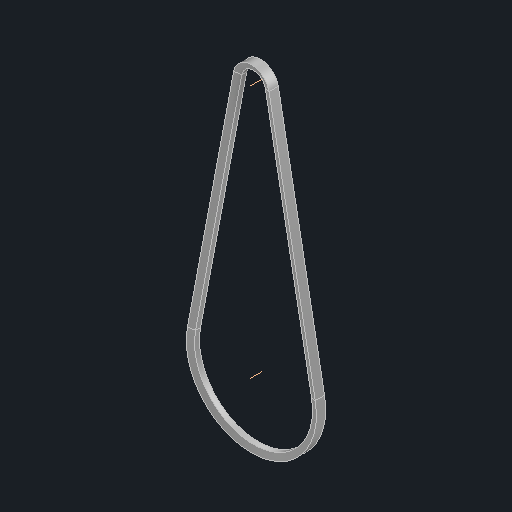
# Autodesk Inventor part: Courroie trapézoïdale
Saved by Autodesk Inventor 2026.2 (Build 302298010, 298A)
## iProperties
CustomPartVersion: 1
Created: 2026-03-31
Part Number: Courroie trapézoïdale
Material: Rubber
Document SubType Name: Modeling
Designer: romai
Density: 0.93 g/cm^3
Appearance: Rubber - Black - Version 1.1
Author: romai
Autodesk Inventor part; units mm, degrees
ref_plane "YZ Plane" through (0, 0, 0) normal (1, 0, 0) x (0, 1, 0)
ref_plane "XZ Plane" through (0, 0, 0) normal (0, 1, 0) x (-1, 0, 0)
sketch "Chemin d'esquisse" plane through (0, 0, 0) normal (0, 0, 1) x (1, 0, 0)
  arc A0 (-112.5064, 21.2735) -> (112.5064, 21.2735) centre (0, 0) ccw
  arc A1 (28.1512, 467.393) -> (-28.1512, 467.393) centre (0, 462.07) ccw
  line L0 (28.1512, 467.393) -> (112.5064, 21.2735)
  line L1 (-112.5064, 21.2735) -> (-28.1512, 467.393)
  constraints: 4 end point, 4 point on circle, 2 centre point
ref_plane "Plan de section" through (112.5064, 21.2735, 0) normal (-0.1858, 0.9826, 0) x (0, 0, 1)
sketch "Section" plane through (112.5064, 21.2735, 0) normal (-0.1858, 0.9826, 0) x (0, 0, 1)
  line L0 (0, 4.1563) -> (0, -6.8437) construction
  line L1 (-7, 0) -> (7, 0) construction
  line L2 (-8.5128, 4.1563) -> (8.5128, 4.1563)
  line L3 (8.5128, 4.1563) -> (4.5091, -6.8437)
  line L4 (4.5091, -6.8437) -> (-4.5091, -6.8437)
  line L5 (-4.5091, -6.8437) -> (-8.5128, 4.1563)
  point P0 (0, 0)
  point P1 (0, 0)
  point P2 (0, 0)
  dimension "d0" = 14
  dimension "d1" = 4.1563
  dimension "d2" = 40
  dimension "d3" = 11
  constraints: 12 end point, 3 midpoint, 2 parallel, 2 point on line, 1 coincident, 1 perpendicular, 1 vertical, 1 other
  measures "d0" distance of L1.start L1.end
  measures "d1" distance between parallel lines of L2 L1
  measures "d2" angle of L5 L3
  measures "d3" distance between parallel lines of L4 L2
sweep "Courroie" add profiles "Section" path "Chemin d'esquisse"
equation "\"d0\" = da_Bw"
equation "\"d1\" = da_Hw"
equation "\"d2\" = da_Alfa"
equation "\"d3\" = da_H"
equation "\"da_Alfa\" = 40deg"
equation "\"da_H\" = 11"
equation "\"da_Bw\" = 14"
equation "\"da_Hw\" = 4.15634"
body "Solid1"
